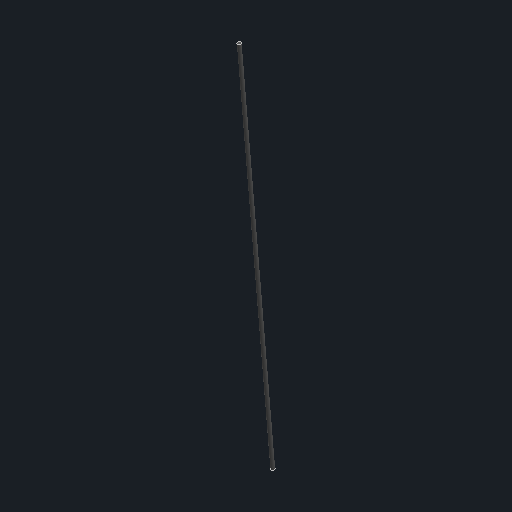
# Autodesk Inventor part: steering_rod
Saved by Autodesk Inventor 2022.2 (Build 262287010, 287A)
## iProperties
Created: 2022-03-30
Part Number: steering_rod
Material: Generic
Document SubType Name: Modeling
Designer: kardo
Density: 1 g/cm^3
Appearance: Dark Plastic
Author: kardo
Autodesk Inventor part; units mm, degrees
ref_plane "YZ Plane" through (0, 0, 0) normal (1, 0, 0) x (0, 1, 0)
ref_plane "XZ Plane" through (0, 0, 0) normal (0, 1, 0) x (-1, 0, 0)
ref_plane "XY Plane" through (0, 0, 0) normal (0, 0, 1) x (1, 0, 0)
derived "stencil_frame.ipt"
sketch3d "sk_servo_rod"
ref_plane "Work Plane1" through (-19.6, -191.0082, 43.6084) normal (0.0026932, -0.9964437, -0.084218) x (0.9999963, 0.0027028, 0)
sketch "Sketch1" plane through (-19.6, -191.0082, 43.6084) normal (0.0026932, -0.9964437, -0.084218) x (0.9999963, 0.0027028, 0)
  circle A0 centre (0, 0) radius 1
  point P0 (20.1162, -59.5353)
  point P1 (0, 0)
  dimension "d1" = 2
  constraints: 1 centre point, 1 coincident
  measures "d1" diameter of A0
extrude "Extrusion1" add sketch "Sketch1" along normal up to surface (222.7841 mm away)
body "Solid1"
